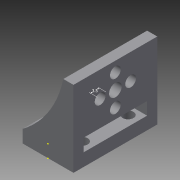
# Autodesk Inventor part: PickJoint
Saved by Autodesk Inventor 2015 (Build 190159000, 159)
## iProperties
Created: 2016-04-24
Part Number: PickJoint
Material: Generic
Document SubType Name: Modeling
Designer: Hatch
Density: 1 g/cm^3
Appearance: Default
Author: Hatch
Autodesk Inventor part; units mm, degrees
ref_plane "YZ Plane" through (0, 0, 0) normal (1, 0, 0) x (0, 1, 0)
ref_plane "XZ Plane" through (0, 0, 0) normal (0, 1, 0) x (-1, 0, 0)
ref_plane "XY Plane" through (0, 0, 0) normal (0, 0, 1) x (1, 0, 0)
sketch "Sketch1" plane through (0, 0, 0) normal (0, 1, 0) x (-1, 0, 0)
  circle A0 centre (0, 0) radius 10
  dimension "d0" = 20
  constraints: 1 centre point, 1 coincident
  measures "d0" diameter of A0
extrude "Extrusion1" add sketch "Sketch1" along normal blind 4
sketch "Sketch2" plane through (0, 4, 0) normal (0, 1, 0) x (1, 0, 0)
  line L0 (0, 0) -> (0, 6)
  circle A0 centre (0, 6) radius 2.125
  dimension "d3" = 6
  dimension "d4" = 4.25
  constraints: 2 end point, 1 centre point, 1 coincident, 1 vertical
  measures "d3" distance of L0.start L0.end
  measures "d4" diameter of A0
extrude "Extrusion2" cut sketch "Sketch2" against normal through all
pattern_circular "Circular Pattern1" count 4 over 360 about axis through (0, 0, 0) along (0, 1, 0) of "Extrusion2"
sketch "Sketch3" plane through (0, 0, 0) normal (0, -1, 0) x (1, 0, 0)
  circle A0 centre (0, 0) radius 10 projected
  arc A1 (-10, 0) -> (10, 0) centre (0, 0) ccw
  line L0 (10, 0) -> (10, -25)
  line L1 (10, -25) -> (-10, -25)
  line L2 (-10, -25) -> (-10, 0)
  dimension "d10" = 25
  constraints: 6 end point, 2 perpendicular, 2 point on circle, 2 tangent, 2 vertical, 1 centre point, 1 horizontal alignment, 1 other
  measures "d10" distance of L0.start L0.end
extrude "Extrusion3" add sketch "Sketch3" against normal blind 4 contours L0 L1 L2 A0
sketch "Sketch4" plane through (0, 4, 0) normal (0, 1, 0) x (1, 0, 0)
  line L0 (-10, 25) -> (-10, 0) projected
  line L1 (10, 25) -> (-10, 25)
  line L2 (-10, 25) -> (-10, 20)
  line L3 (-10, 20) -> (10, 20)
  line L4 (10, 20) -> (10, 25)
  point P0 (0, 0)
  dimension "d13" = 5
  constraints: 8 end point, 2 parallel, 1 horizontal, 1 perpendicular, 1 point on line
  measures "d13" distance of L2.end L1.end
extrude "Extrusion4" add sketch "Sketch4" along normal blind 27
sketch "Sketch5" plane through (10, 0, -25) normal (0, 0, -1) x (-1, 0, 0)
  point P0 (10, 0)
sketch "Sketch6" plane through (10, 0, -25) normal (0, 0, -1) x (-1, 0, 0)
  line L0 (7.875, 4) -> (12.125, 4) projected
  line L1 (20, 31) -> (0, 31) projected
  line L2 (10, 17.5) -> (20, 17.5)
  line L3 (10, 17.5) -> (10, 23.5)
  line L4 (10, 23.5) -> (10, 25.5)
  circle A0 centre (10, 25.5) radius 2.125
  point P0 (10, 0)
  dimension "d16" = 6
  dimension "d26" = 2
  dimension "d27" = 4.25
  constraints: 6 end point, 2 coincident, 1 centre point, 1 horizontal, 1 vertical
  measures "d16" distance of L2.start L3.end
  measures "d26" distance of L4.start L4.end
  measures "d27" diameter of A0
extrude "Extrusion5" cut sketch "Sketch6" against normal through all
pattern_linear "Rectangular Pattern1" count 3 spacing 6 along (-1, 0, 0) count 2 spacing 18 along (0, -1, 0) of "Extrusion5" first direction both ways yes
sketch "Sketch7" plane through (-10, 4, -20) normal (0, 0, 1) x (1, 0, 0)
  circle A0 centre (10, 21.5) radius 2.125 projected
  circle A1 centre (10, 3.5) radius 2.125 projected
  line L0 (10, 21.5) -> (10, 3.5)
  line L1 (6, 7) -> (14, 7)
  line L2 (14, 7) -> (14, 18)
  line L3 (14, 18) -> (6, 18)
  line L4 (6, 18) -> (6, 7)
  line L5 (6, 7) -> (14, 18) construction
  line L6 (14, 7) -> (6, 18) construction
  point P0 (10, -4)
  point P1 (10, 12.5)
  dimension "d29" = 8
  dimension "d30" = 11
  constraints: 14 end point, 3 midpoint, 2 parallel, 1 horizontal, 1 perpendicular, 1 vertical
  measures "d29" distance of L3.end L2.end
  measures "d30" distance of L2.end L1.end
extrude "Extrusion6" cut sketch "Sketch7" against normal through all contours L3 L2 L1 L0 | L0 L1 L4 L3
sketch "Sketch8" plane through (-10, 4, -20) normal (0, 0, 1) x (1, 0, 0)
  circle A0 centre (4, 21.5) radius 2.125 projected
  line L0 (4, 21.5) -> (4, 25)
  point P0 (10, -4)
  dimension "d33" = 3.5
  constraints: 2 end point, 1 vertical
  measures "d33" distance of L0.start L0.end
sketch "Sketch9" plane through (10, 0, -25) normal (0, 0, -1) x (-1, 0, 0)
  circle A0 centre (16, 25.5) radius 2.125 projected
  line L0 (16, 25.5) -> (16, 29)
  line L1 (20, 4) -> (20, 31) projected
  line L2 (20, 29) -> (0, 29)
  line L3 (0, 29) -> (0, 33)
  line L4 (0, 33) -> (20, 33)
  line L5 (20, 33) -> (20, 29)
  point P0 (10, 0)
  dimension "d34" = 3.5
  dimension "d35" = 4
  constraints: 10 end point, 2 parallel, 1 horizontal, 1 perpendicular, 1 point on line, 1 vertical
  measures "d34" distance of L0.start L0.end
  measures "d35" distance of L2.end L3.end
extrude "Extrusion7" add sketch "Sketch9" against normal blind 30 contours L2 L3 L4 L5 L1
sketch "Sketch10" plane through (0, 0, 0) normal (0, -1, 0) x (1, 0, 0)
  line L0 (-10, -20) -> (11.4929, -20)
  line L1 (11.4929, -20) -> (11.4929, 11.4929)
  line L2 (11.4929, 11.4929) -> (-10, 11.4929)
  line L3 (-10, 11.4929) -> (-10, -20)
  point P0 (0, 0)
  constraints: 8 end point, 2 parallel, 1 horizontal, 1 perpendicular
extrude "Extrusion8" cut sketch "Sketch10" against normal blind 4
sketch "Sketch11" plane through (-10, 0, -20) normal (0, 0, 1) x (1, 0, 0)
  line L0 (20, 29) -> (20, 0) projected
  line L1 (0, 0) -> (20, 0)
  line L2 (20, 0) -> (20, 4)
  line L3 (20, 4) -> (0, 4)
  line L4 (0, 4) -> (0, 0)
  point P0 (10, 0)
  dimension "d40" = 4
  constraints: 8 end point, 2 parallel, 1 horizontal, 1 perpendicular, 1 point on line
  measures "d40" distance of L2.end L1.end
extrude "Extrusion9" add sketch "Sketch11" along normal blind 25
sketch "Sketch12" plane through (10, 0, -25) normal (1, 0, 0) x (0, 0, -1)
  line L0 (-5, 29) -> (-30, 29) projected
  line L1 (-30, 4) -> (-10, 4)
  line L2 (-10, 4) -> (-10, 29)
  line L3 (-10, 29) -> (-30, 29)
  line L4 (-30, 29) -> (-30, 4)
  point P0 (-25, 0)
  dimension "d43" = 20
  constraints: 8 end point, 2 parallel, 1 horizontal, 1 perpendicular, 1 point on line
  measures "d43" distance of L3.end L2.end
extrude "Extrusion10" add sketch "Sketch12" against normal blind 4
sketch "Sketch13" plane through (10, 0, 5) normal (1, 0, 0) x (0, 0, -1)
  line L0 (20, 29) -> (20, 4) projected
  line L1 (20, 16.5) -> (0, 16.5)
  line L2 (0, 0) -> (0, 33) projected
  line L3 (10, 16.5) -> (4, 16.5)
  circle A0 centre (10, 16.5) radius 2.5
  point P0 (5, 0)
  dimension "d46" = 6
  dimension "d47" = 5
  constraints: 4 end point, 3 midpoint, 1 centre point, 1 coincident, 1 point on line
  measures "d46" distance of L3.start L3.end
  measures "d47" diameter of A0
extrude "Extrusion11" cut sketch "Sketch13" against normal through all
sketch "Sketch14" plane through (10, 0, 5) normal (1, 0, 0) x (0, 0, -1)
  circle A0 centre (10, 16.5) radius 2.5 projected
  line L0 (10, 16.5) -> (4, 16.5)
  circle A1 centre (4, 16.5) radius 2.125
  point P0 (5, 0)
  dimension "d50" = 6
  dimension "d51" = 4.25
  constraints: 2 end point, 1 centre point, 1 coincident, 1 horizontal
  measures "d50" distance of L0.start L0.end
  measures "d51" diameter of A1
extrude "Extrusion12" cut sketch "Sketch14" against normal through all contours A1
pattern_circular "Circular Pattern2" count 4 over 360 about axis through (10, 16.5, -5) along (-1, 0, 0) of "Extrusion12"
sketch "Sketch15" plane through (-10, 33, -25) normal (0, 1, 0) x (1, 0, 0)
  line L0 (16, -30) -> (0, -30)
  line L1 (0, -30) -> (16, -30) projected
  line L2 (0, -30) -> (0, -5)
  line L3 (0, 0) -> (0, -30) projected
  arc A0 (16, -30) -> (0, -5) centre (-25.4317, -38.8963) ccw
  point P0 (10, -25)
  dimension "d57" = 25
  constraints: 4 end point, 2 point on circle, 1 centre point, 1 collinear, 1 point on line
  measures "d57" distance of L0.end L2.end
extrude "Extrusion13" cut sketch "Sketch15" against normal through all
body "Solid1"
